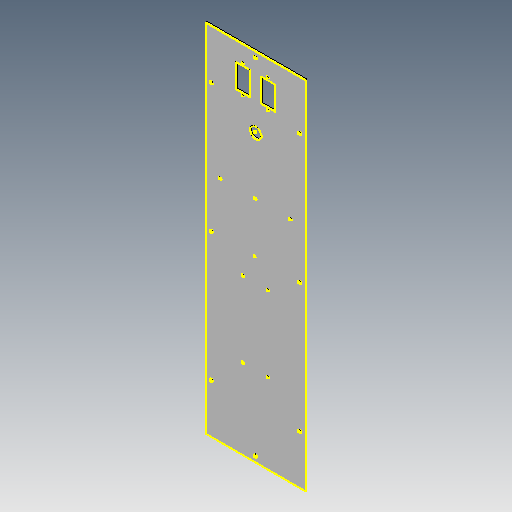
# Autodesk Inventor part: Cut_A
Saved by Autodesk Inventor 2020 (Build 240168000, 168)
## iProperties
Created: 2021-12-11
Part Number: Cut_A
Material: Generic
Document SubType Name: Modeling
Designer: magnarecta
Density: 1 g/cm^3
Appearance: Default
Author: magnarecta
Autodesk Inventor part; units mm, degrees
ref_plane "YZ Plane" through (0, 0, 0) normal (1, 0, 0) x (0, 1, 0)
ref_plane "XZ Plane" through (0, 0, 0) normal (0, 1, 0) x (-1, 0, 0)
ref_plane "XY Plane" through (0, 0, 0) normal (0, 0, 1) x (1, 0, 0)
sketch "スケッチ1" plane through (0, 0, 0) normal (0, 0, 1) x (1, 0, 0)
  line L0 (99, -354) -> (-99, -354)
  line L1 (-99, -354) -> (-99, 354)
  line L2 (-99, 354) -> (99, 354)
  line L3 (99, 354) -> (99, -354)
  line L4 (99, -354) -> (-99, 354) construction
  line L5 (-99, -354) -> (99, 354) construction
  point P0 (0, 0)
  dimension "d0" = 198
  dimension "d1" = 708
  constraints: 12 end point, 2 midpoint, 2 parallel, 1 horizontal, 1 perpendicular
  measures "d0" distance of L1.end L2.end
  measures "d1" distance of L0.end L1.end
extrude "押し出し1" add sketch "スケッチ1" along normal blind 3
sketch "スケッチ4" plane through (0, 0, 0) normal (0, 0, -1) x (-1, 0, 0)
  line L0 (99, -354) -> (-99, -354) projected
  line L1 (99, 354) -> (99, -354) projected
  line L2 (-99, 354) -> (99, 354) projected
  line L3 (-99, -354) -> (-99, 354) projected
  line L4 (-88, 343) -> (88, 343)
  line L5 (88, 343) -> (88, -343)
  line L6 (88, -343) -> (-88, -343)
  line L7 (-88, -343) -> (-88, 343)
  line L8 (-88, -256.5) -> (88, -256.5)
  line L9 (88, -256.5) -> (88, 256.5)
  line L10 (88, 256.5) -> (-88, 256.5)
  line L11 (-88, 256.5) -> (-88, -256.5)
  point P0 (0, 0)
  point P1 (0, -343)
  point P2 (0, 343)
  point P3 (-88, 0)
  point P4 (88, 0)
  dimension "d32" = 11
  dimension "d33" = 86.5
  dimension "d34" = 86.5
  constraints: 16 end point, 4 midpoint, 2 parallel, 2 point on line, 1 horizontal, 1 perpendicular, 3 other
  measures "d32" distance between parallel lines of L3 L7
  measures "d33" distance from line of L8 point (0, -343)
  measures "d34" distance from line of point (0, 343) L10
hole "穴3" at (0, -343, 0) at (0, 343, 0) at (88, 0, 0) at (-88, 0, 0) at (-88, -256.5, 0) at (88, -256.5, 0) at (88, 256.5, 0) at (-88, 256.5, 0) direction (0, 0, 1) diameter 6 end through all
sketch "スケッチ5" plane through (0, 0, 3) normal (0, 0, 1) x (1, 0, 0)
  circle A0 centre (88, 256.5) radius 3 projected
  circle A1 centre (-88, -256.5) radius 3 projected
  circle A2 centre (88, 0) radius 3 projected
  circle A3 centre (0, -343) radius 3 projected
  circle A4 centre (0, 343) radius 3 projected
  circle A5 centre (-88, 0) radius 3 projected
  circle A6 centre (88, -256.5) radius 3 projected
  circle A7 centre (-88, 256.5) radius 3 projected
  line L0 (-99, -354) -> (99, -354) projected
  line L1 (99, -354) -> (99, 354) projected
  line L2 (99, 354) -> (-99, 354) projected
  line L3 (-99, 354) -> (-99, -354) projected
  line L4 (-25, -45) -> (25, -45)
  line L5 (25, -45) -> (25, -195)
  line L6 (25, -195) -> (-25, -195)
  line L7 (-25, -195) -> (-25, -45)
  line L8 (-25, -45) -> (25, -195) construction
  line L9 (25, -45) -> (-25, -195) construction
  point P0 (0, 0)
  point P1 (0, -120)
  point P2 (0, -120)
  dimension "d42" = 150
  dimension "d43" = 50
  dimension "d44" = 120
  constraints: 12 end point, 3 midpoint, 2 parallel, 1 horizontal, 1 perpendicular, 1 vertical alignment
  measures "d42" distance of L4.end L5.end
  measures "d43" distance of L5.end L6.end
  measures "d44" distance of point (0, -120) point (0, 0)
hole "穴4" at (-25, -45, 3) at (25, -45, 3) at (-25, -195, 3) at (25, -195, 3) direction (0, 0, -1) diameter 4.2 end through all
sketch "スケッチ6" plane through (0, 0, 3) normal (0, 0, 1) x (1, 0, 0)
  circle A0 centre (-25, -195) radius 2.1 projected
  circle A1 centre (-25, -45) radius 2.1 projected
  circle A2 centre (25, -45) radius 2.1 projected
  circle A3 centre (25, -195) radius 2.1 projected
  circle A4 centre (88, 256.5) radius 3 projected
  circle A5 centre (-88, -256.5) radius 3 projected
  circle A6 centre (88, 0) radius 3 projected
  circle A7 centre (0, -343) radius 3 projected
  circle A8 centre (0, 343) radius 3 projected
  circle A9 centre (-88, 0) radius 3 projected
  circle A10 centre (88, -256.5) radius 3 projected
  circle A11 centre (-88, 256.5) radius 3 projected
  line L0 (-99, -354) -> (99, -354) projected
  line L1 (99, -354) -> (99, 354) projected
  line L2 (99, 354) -> (-99, 354) projected
  line L3 (-99, 354) -> (-99, -354) projected
  line L4 (11, 316.5) -> (39, 316.5)
  line L5 (39, 316.5) -> (39, 269.5)
  line L6 (39, 269.5) -> (11, 269.5)
  line L7 (11, 269.5) -> (11, 316.5)
  line L8 (11, 316.5) -> (39, 269.5) construction
  line L9 (39, 316.5) -> (11, 269.5) construction
  line L10 (-39, 316.5) -> (-11, 316.5)
  line L11 (-11, 316.5) -> (-11, 269.5)
  line L12 (-11, 269.5) -> (-39, 269.5)
  line L13 (-39, 269.5) -> (-39, 316.5)
  line L14 (-39, 316.5) -> (-11, 269.5) construction
  line L15 (-11, 316.5) -> (-39, 269.5) construction
  line L16 (25, 321) -> (-25, 321)
  line L17 (-25, 321) -> (-25, 265)
  line L18 (-25, 265) -> (25, 265)
  line L19 (25, 265) -> (25, 321)
  circle A12 centre (25, 321) radius 1.6
  circle A13 centre (25, 265) radius 1.6
  circle A14 centre (-25, 265) radius 1.6
  circle A15 centre (-25, 321) radius 1.6
  point P0 (0, 0)
  point P1 (25, 293)
  point P2 (-25, 293)
  point P3 (-25, 293)
  point P4 (25, 293)
  point P5 (-25, 293)
  point P6 (25, 293)
  point P7 (-23.4, 265)
  point P8 (-25, 266.6)
  dimension "d52" = 47
  dimension "d53" = 28
  dimension "d54" = 28
  dimension "d55" = 50
  dimension "d56" = 25
  dimension "d57" = 50
  dimension "d58" = 56
  dimension "d59" = 28
  dimension "d60" = 3.2
  dimension "d61" = 3.2
  dimension "d62" = 3.2
  dimension "d63" = 3.2
  constraints: 32 end point, 8 midpoint, 6 parallel, 4 centre point, 4 coincident, 3 horizontal, 3 perpendicular, 2 horizontal alignment, 2 vertical alignment
  measures "d52" distance of L4.end L5.end
  measures "d53" distance of L5.end L6.end
  measures "d54" distance of L11.end L12.end
  measures "d55" distance of point (25, 293) point (-25, 293)
  measures "d56" horizontal distance of point (25, 293) A8.centre
  measures "d57" vertical distance of point (25, 293) A8.centre
  measures "d58" distance of L16.end L17.end
  measures "d59" distance from line of L18 point (25, 293)
  measures "d60" diameter of A12
  measures "d61" diameter of A13
  measures "d62" diameter of A14
  measures "d63" diameter of A15
extrude "押し出し2" cut sketch "スケッチ6" against normal blind 10 contours L4 L19 L6 L7 | L4 L5 L6 L19 | A12 L16 L19 | L19 L16 A12 | A13 L18 L19 | L19 L18 A13 | A15 L17 L16 | L16 L17 A15 | A14 L17 L18 | L18 L17 A14 | L17 L12 L13 L10 | L10 L11 L12 L17
sketch "スケッチ7" plane through (0, 0, 3) normal (0, 0, 1) x (1, 0, 0)
  circle A0 centre (0, 214) radius 11.15
  line L0 (99, 354) -> (-99, 354) projected
  point P0 (0, 0)
  dimension "d66" = 22.3
  dimension "d67" = 140
  constraints: 1 centre point, 1 vertical alignment
  measures "d66" diameter of A0
  measures "d67" distance from line of A0.centre L0
extrude "押し出し3" cut sketch "スケッチ7" against normal blind 10
sketch "スケッチ8" plane through (0, 0, 3) normal (0, 0, 1) x (1, 0, 0)
  line L0 (4.8167, 215.6) -> (13.35, 215.6)
  line L1 (13.35, 215.6) -> (13.35, 212.4)
  line L2 (13.35, 212.4) -> (4.8167, 212.4)
  line L3 (4.8167, 212.4) -> (4.8167, 215.6)
  circle A0 centre (0, 214) radius 11.15 projected
  circle A1 centre (0, 214) radius 11.15 projected
  point P0 (0, 0)
  point P1 (-11.15, 214)
  point P2 (11.0346, 215.6)
  point P3 (11.0346, 212.4)
  dimension "d70" = 3.2
  dimension "d71" = 1.6
  dimension "d72" = 24.5
  constraints: 8 end point, 2 parallel, 1 horizontal, 1 horizontal alignment, 1 perpendicular, 1 other
  measures "d70" distance of L0.end L1.end
  measures "d71" distance from line of A0.centre L0
  measures "d72" distance from line of L1 point (-11.15, 214)
extrude "押し出し4" cut sketch "スケッチ8" against normal blind 10 contours L0 L1 L2 A0
sketch "スケッチ9" plane through (0, 0, 3) normal (0, 0, 1) x (1, 0, 0)
  point P0 (0, 0)
  point P1 (70, 100)
  point P2 (-70, 100)
  point P3 (0, 100)
  dimension "d75" = 140
  dimension "d76" = 70
  dimension "d77" = 100
  constraints: 2 horizontal alignment, 1 vertical alignment
  measures "d75" distance of point (-70, 100) point (70, 100)
  measures "d76" horizontal distance of point (0, 0) point (70, 100)
  measures "d77" vertical distance of point (-70, 100) point (0, 0)
hole "穴5" at (70, 100, 3) at (-70, 100, 3) at (0, 100, 3) direction (0, 0, -1) diameter 4.2 end through all
sketch "スケッチ10" plane through (0, 0, 3) normal (0, 0, 1) x (1, 0, 0)
  circle A0 centre (-70, 100) radius 2.1 projected
  circle A1 centre (70, 100) radius 2.1 projected
  circle A2 centre (0, 100) radius 2.1 projected
  line L0 (13.35, 212.4) -> (11.0346, 212.4) projected
  arc A3 (11.0346, 215.6) -> (11.0346, 212.4) centre (0, 214) ccw projected
  line L1 (11.0346, 215.6) -> (13.35, 215.6) projected
  line L2 (13.35, 215.6) -> (13.35, 212.4) projected
  circle A4 centre (25, 265) radius 1.6 projected
  line L3 (11, 269.5) -> (11, 316.5) projected
  line L4 (11, 316.5) -> (39, 316.5) projected
  line L5 (39, 316.5) -> (39, 269.5) projected
  line L6 (39, 269.5) -> (11, 269.5) projected
  circle A5 centre (-25, 321) radius 1.6 projected
  circle A6 centre (-25, 265) radius 1.6 projected
  circle A7 centre (25, 321) radius 1.6 projected
  line L7 (-11, 269.5) -> (-39, 269.5) projected
  line L8 (-39, 269.5) -> (-39, 316.5) projected
  line L9 (-39, 316.5) -> (-11, 316.5) projected
  line L10 (-11, 316.5) -> (-11, 269.5) projected
  circle A8 centre (-25, -195) radius 2.1 projected
  circle A9 centre (-25, -45) radius 2.1 projected
  circle A10 centre (25, -45) radius 2.1 projected
  circle A11 centre (25, -195) radius 2.1 projected
  circle A12 centre (88, 256.5) radius 3 projected
  circle A13 centre (-88, -256.5) radius 3 projected
  circle A14 centre (88, 0) radius 3 projected
  circle A15 centre (0, -343) radius 3 projected
  circle A16 centre (0, 343) radius 3 projected
  circle A17 centre (-88, 0) radius 3 projected
  circle A18 centre (88, -256.5) radius 3 projected
  circle A19 centre (-88, 256.5) radius 3 projected
  line L11 (-99, -354) -> (99, -354) projected
  line L12 (99, -354) -> (99, 354) projected
  line L13 (99, 354) -> (-99, 354) projected
  line L14 (-99, 354) -> (-99, -354) projected
  point P0 (0, 0)
